Autodesk Inventor part; units mm, degrees
note: some values were not read from the file. Chosen so that the rebuilt part matches the saved one: direction of "Hole2".
(part 14 of 20)
  spline S82 degree 3 poles (-108.596575, -51.704661) (-108.591829, -51.705287) (-108.581504, -51.706647) (-108.566848, -51.71629) (-108.552275, -51.730819) (-108.537912, -51.751139) (-108.524031, -51.776791) (-108.505397, -51.819556) (-108.489595, -51.868576) (-108.475979, -51.923076) (-108.46262, -51.987447) (-108.449286, -52.075757) (-108.439921, -52.186978) (-108.436583, -52.301561) (-108.439921, -52.416145) (-108.449286, -52.527366) (-108.46262, -52.615676) (-108.475979, -52.680047) (-108.489595, -52.734547) (-108.505397, -52.783567) (-108.524031, -52.826332) (-108.537912, -52.851984) (-108.552275, -52.872304) (-108.566848, -52.886832) (-108.581504, -52.896476) (-108.591829, -52.897836) (-108.596575, -52.898461) knots 0 0 0 0 0.01106677 0.02407754 0.03992786 0.05913986 0.0819337 0.10802006 0.16805875 0.20201508 0.23929564 0.3216678 0.41056278 0.5 0.58943722 0.6783322 0.76070436 0.79798492 0.83194125 0.89197994 0.9180663 0.94086014 0.96007214 0.97592246 0.98893323 1 1 1 1
  spline S83 degree 3 poles (-108.596575, -52.898461) (-108.601237, -52.897852) (-108.611254, -52.896542) (-108.62517, -52.886862) (-108.638409, -52.872259) (-108.65094, -52.851903) (-108.662566, -52.826236) (-108.677691, -52.783344) (-108.689782, -52.734349) (-108.699832, -52.679969) (-108.709479, -52.61551) (-108.718735, -52.527157) (-108.725048, -52.416046) (-108.727236, -52.301561) (-108.725048, -52.187077) (-108.718735, -52.075966) (-108.709479, -51.987613) (-108.699832, -51.923154) (-108.689782, -51.868774) (-108.677691, -51.819779) (-108.662566, -51.776887) (-108.65094, -51.75122) (-108.638409, -51.730864) (-108.62517, -51.716261) (-108.611254, -51.706581) (-108.601237, -51.705271) (-108.596575, -51.704661) knots 0 0 0 0 0.01099744 0.02362844 0.03895388 0.0576141 0.07990846 0.10559498 0.1652091 0.19914929 0.2365432 0.31951534 0.40940333 0.5 0.59059667 0.68048466 0.7634568 0.80085071 0.8347909 0.89440502 0.92009154 0.9423859 0.96104612 0.97637156 0.98900256 1 1 1 1
  spline S84 degree 3 poles (-85.406507, -52.898461) (-85.411253, -52.897836) (-85.421579, -52.896476) (-85.436235, -52.886832) (-85.450807, -52.872304) (-85.46517, -52.851984) (-85.479051, -52.826332) (-85.497685, -52.783567) (-85.513487, -52.734547) (-85.527103, -52.680047) (-85.540462, -52.615676) (-85.553796, -52.527366) (-85.563161, -52.416145) (-85.566499, -52.301561) (-85.563161, -52.186978) (-85.553796, -52.075757) (-85.540462, -51.987447) (-85.527103, -51.923076) (-85.513487, -51.868576) (-85.497685, -51.819556) (-85.479051, -51.776791) (-85.46517, -51.751139) (-85.450807, -51.730819) (-85.436235, -51.71629) (-85.421579, -51.706647) (-85.411253, -51.705287) (-85.406507, -51.704661) knots 0 0 0 0 0.01106677 0.02407754 0.03992786 0.05913986 0.0819337 0.10802006 0.16805875 0.20201508 0.23929564 0.3216678 0.41056278 0.5 0.58943722 0.6783322 0.76070436 0.79798492 0.83194125 0.89197994 0.9180663 0.94086014 0.96007214 0.97592246 0.98893323 1 1 1 1
  spline S85 degree 3 poles (-85.406507, -51.704661) (-85.401845, -51.705271) (-85.391828, -51.706581) (-85.377912, -51.716261) (-85.364673, -51.730864) (-85.352142, -51.75122) (-85.340516, -51.776887) (-85.325391, -51.819779) (-85.3133, -51.868774) (-85.30325, -51.923154) (-85.293603, -51.987613) (-85.284347, -52.075966) (-85.278034, -52.187077) (-85.275846, -52.301561) (-85.278034, -52.416046) (-85.284347, -52.527157) (-85.293603, -52.61551) (-85.30325, -52.679969) (-85.3133, -52.734349) (-85.325391, -52.783344) (-85.340516, -52.826236) (-85.352142, -52.851903) (-85.364673, -52.872259) (-85.377912, -52.886862) (-85.391828, -52.896542) (-85.401845, -52.897852) (-85.406507, -52.898461) knots 0 0 0 0 0.01099744 0.02362844 0.03895388 0.0576141 0.07990846 0.10559498 0.1652091 0.19914929 0.2365432 0.31951534 0.40940333 0.5 0.59059667 0.68048466 0.7634568 0.80085071 0.8347909 0.89440502 0.92009154 0.9423859 0.96104612 0.97637156 0.98900256 1 1 1 1
  line L1833 (-101.214785, -54.709561) -> (-101.214785, -54.801561)
  line L1834 (-106.155772, -54.801561) -> (-106.155772, -54.201561)
  line L1835 (-101.214785, -54.801561) -> (-106.155772, -54.801561)
  line L1836 (-92.788297, -54.801561) -> (-92.788297, -54.709561)
  line L1837 (-87.84731, -54.801561) -> (-92.788297, -54.801561)
  line L1838 (-87.84731, -54.201561) -> (-87.84731, -54.801561)
  line L1839 (-101.001541, -54.201561) -> (-106.155772, -54.201561)
  line L1840 (-87.84731, -54.201561) -> (-93.001541, -54.201561)
  line L1841 (-85.051541, -54.801561) -> (-87.84731, -54.801561)
  line L1842 (-106.155772, -54.801561) -> (-108.951541, -54.801561)
  line L1843 (-93.001541, -49.801561) -> (-85.051541, -49.801561)
  line L1844 (-108.951541, -49.801561) -> (-101.001541, -49.801561)
  line L1845 (-108.951541, -54.801561) -> (-108.951541, -49.801561)
  line L1846 (-85.051541, -54.801561) -> (-85.051541, -49.801561)
  line L1847 (-92.788297, -54.801561) -> (-93.098156, -54.801561)
  line L1848 (-93.098156, -54.801561) -> (-93.098156, -54.709561)
  line L1849 (-93.098156, -54.801561) -> (-101.214785, -54.801561)
  line L1850 (-106.083905, -39.801561) -> (-100.326678, -39.801561)
  line L1851 (-93.676404, -39.801561) -> (-87.919177, -39.801561)
  line L1852 (-86.351309, -39.801561) -> (-85.788245, -39.801561)
  line L1853 (-108.214837, -39.801561) -> (-107.651773, -39.801561)
  line L1854 (-85.788245, -49.801561) -> (-85.788245, -39.801561)
  line L1855 (-108.214837, -39.801561) -> (-108.214837, -49.801561)
  spline S86 degree 3 poles (-105.769333, -47.200601) (-105.769074, -47.090365) (-105.765671, -46.866439) (-105.74757, -46.534003) (-105.717423, -46.260803) (-105.684088, -46.071483) (-105.649602, -45.979267) (-105.626193, -45.9168) (-105.576966, -45.914333) (-105.549364, -45.954376) (-105.514531, -46.034958) (-105.477403, -46.221178) (-105.445921, -46.494501) (-105.427985, -46.825972) (-105.423589, -47.159297) (-105.431148, -47.492218) (-105.451141, -47.826101) (-105.483037, -48.098141) (-105.518843, -48.287815) (-105.551255, -48.379074) (-105.575083, -48.444765) (-105.624435, -48.444965) (-105.650788, -48.40348) (-105.681562, -48.322842) (-105.718652, -48.137084) (-105.747883, -47.864653) (-105.76544, -47.532488) (-105.76959, -47.309883) (-105.769333, -47.200601) knots 0 0 0 0 0.06370705 0.12949472 0.19191208 0.22368799 0.2382902 0.25135028 0.25660425 0.26301775 0.27714857 0.30853838 0.37103998 0.43687849 0.50002298 0.56369496 0.62938323 0.69283553 0.72316052 0.73857311 0.75180992 0.75696152 0.7632602 0.77795176 0.80804313 0.87131401 0.93684349 1 1 1 1
  spline S87 degree 3 poles (-107.965507, -47.119008) (-107.964893, -46.896289) (-107.954528, -46.572436) (-107.954488, -46.176033) (-107.916737, -46.017933) (-107.925964, -45.924139) (-107.889328, -45.914097) (-107.8786, -45.994541) (-107.86006, -46.081863) (-107.845025, -46.30216) (-107.831555, -46.57198) (-107.82423, -46.905828) (-107.820159, -47.352241) (-107.835826, -47.785121) (-107.839355, -48.182231) (-107.879062, -48.341118) (-107.869754, -48.435677) (-107.907095, -48.446175) (-107.915715, -48.363737) (-107.933723, -48.276705) (-107.945951, -48.0556) (-107.962013, -47.678267) (-107.966123, -47.341986) (-107.965507, -47.119008) knots 0 0 0 0 0.13139199 0.19506211 0.22486648 0.236537 0.23877104 0.24363774 0.27264718 0.30298792 0.36807806 0.43503205 0.49911295 0.63103815 0.69471519 0.72474683 0.73665002 0.73889428 0.74387281 0.77307947 0.80345172 0.86845517 1 1 1 1
  spline S88 degree 3 poles (-88.577615, -47.119008) (-88.57729, -47.008677) (-88.574234, -46.78406) (-88.552396, -46.455188) (-88.522944, -46.174531) (-88.475521, -46.007946) (-88.439428, -45.916086) (-88.390424, -45.914818) (-88.347089, -45.976964) (-88.316595, -46.08799) (-88.279777, -46.300167) (-88.252588, -46.57628) (-88.236182, -46.907606) (-88.231986, -47.240889) (-88.239004, -47.574267) (-88.258558, -47.903462) (-88.289101, -48.183006) (-88.332842, -48.350609) (-88.365074, -48.442504) (-88.414556, -48.446229) (-88.458229, -48.380683) (-88.485965, -48.271583) (-88.527334, -48.059183) (-88.5545, -47.78425) (-88.573579, -47.45108) (-88.577937, -47.228226) (-88.577615, -47.119008) knots 0 0 0 0 0.06377364 0.12947571 0.19191728 0.22251596 0.23572674 0.24098241 0.24712107 0.27642984 0.3084167 0.37100213 0.43691035 0.50001881 0.5637377 0.62924964 0.69193924 0.72212339 0.73538665 0.74053978 0.7469427 0.77702751 0.80721947 0.87118814 0.93686953 1 1 1 1
  line L1856 (-87.919177, -39.801561) -> (-86.351309, -39.801561)
  line L1857 (-107.651773, -39.801561) -> (-106.083905, -39.801561)
  spline S89 degree 3 poles (-86.180316, -47.200601) (-86.179625, -46.976697) (-86.177708, -46.642662) (-86.153357, -46.263675) (-86.144704, -46.070685) (-86.121116, -45.985378) (-86.127644, -45.919582) (-86.090265, -45.91624) (-86.086845, -45.961563) (-86.067375, -46.033845) (-86.058579, -46.22558) (-86.044067, -46.494224) (-86.038541, -46.826549) (-86.036712, -47.27203) (-86.040139, -47.717725) (-86.061167, -48.094625) (-86.068571, -48.289359) (-86.090145, -48.371714) (-86.082612, -48.443355) (-86.120246, -48.442499) (-86.123349, -48.396914) (-86.142857, -48.32401) (-86.154386, -48.133195) (-86.177012, -47.757195) (-86.181004, -47.423111) (-86.180316, -47.200601) knots 0 0 0 0 0.13209168 0.19547472 0.22735918 0.24158397 0.25296859 0.25518606 0.26025608 0.27356013 0.30485536 0.36824052 0.43535326 0.4998067 0.63172546 0.69607433 0.72644443 0.74148548 0.75299654 0.75519516 0.76033444 0.77439415 0.80449955 0.86873005 1 1 1 1
  line L1858 (-93.001541, -42.271561) -> (-95.001541, -34.951561)
  line L1859 (-99.001541, -34.951561) -> (-101.001541, -42.271561)
  line L1860 (-93.001541, -53.693561) -> (-93.001541, -42.271561)
  line L1861 (-101.001541, -53.693561) -> (-101.001541, -42.271561)
  line L1862 (-95.001541, -34.951561) -> (-99.001541, -34.951561)
  line L1863 (-93.001541, -53.693561) -> (-93.001541, -54.709561)
  line L1864 (-101.001541, -53.693561) -> (-101.001541, -54.709561)
  line L1865 (-93.001541, -54.709561) -> (-101.001541, -54.709561)
  line L1866 (-105.126509, -54.709561) -> (-105.301369, -54.709561)
  line L1867 (-105.126509, -54.201561) -> (-105.126509, -54.709561)
  line L1868 (-101.424102, -54.709561) -> (-105.126509, -54.709561)
  line L1869 (-101.424102, -54.709561) -> (-101.001541, -54.709561)
  line L1870 (-93.001541, -54.709561) -> (-92.57898, -54.709561)
  line L1871 (-88.876573, -54.709561) -> (-92.57898, -54.709561)
  line L1872 (-88.876573, -54.201561) -> (-88.876573, -54.709561)
  line L1873 (-88.701713, -54.709561) -> (-88.876573, -54.709561)
  line L1874 (-105.301369, -54.201561) -> (-105.301369, -54.709561)
  line L1875 (-88.701713, -54.201561) -> (-88.701713, -54.709561)
  line L1876 (-108.001541, -57.801561) -> (-86.001541, -57.801561)
  line L1877 (-108.001541, -90.801561) -> (-86.001541, -90.801561)
  line L1878 (-108.001541, -90.801561) -> (-108.001541, -57.801561)
  line L1879 (-86.001541, -90.801561) -> (-86.001541, -57.801561)
  line L1880 (-106.400026, -57.801561) -> (-106.400026, -54.801561)
  line L1881 (-104.300026, -57.801561) -> (-104.300026, -54.801561)
  line L1882 (-98.051541, -57.801561) -> (-98.051541, -54.801561)
  line L1883 (-95.951541, -57.801561) -> (-95.951541, -54.801561)
  line L1884 (-89.703056, -57.801561) -> (-89.703056, -54.801561)
  line L1885 (-87.603056, -57.801561) -> (-87.603056, -54.801561)
  point P0 (0, 0)
sketch "Sketch13" plane through (0, 0, 0) normal (1, 0, 0) x (0, 1, 0)
  line L0 (0, -156.78708) -> (0, 91.844197)
  line L1 (0, 25) -> (0, -118.976908)
  line L2 (13.762, 0) -> (-13.762, 0)
  line L3 (-13.762, -15) -> (-13.762, 0)
  line L4 (-0.000559, -82.705424) -> (-0.000559, -41.705424)
  line L5 (6.538534, -24.585438) -> (6.563068, -24.580402)
  ellipse E0 centre (6.661555, -24.562642) end of major axis (7.445275, -24.402071) minor radius 0.002388 (6.818055, -24.52819) -> (6.563068, -24.580402) ccw
  ellipse E1 centre (6.661555, -24.562642) end of major axis (7.445275, -24.402071) minor radius 0.002388 (7.445275, -24.402071) -> (6.993202, -24.492485) ccw
  line L6 (7.445414, -24.402746) -> (7.445275, -24.402071)
  ellipse E2 centre (-6.654323, -24.56163) end of major axis (-7.438018, -24.400939) minor radius 0.002388 (-6.987316, -24.491146) -> (-7.438018, -24.400939) ccw
  line L7 (-5.641341, -24.766384) -> (-5.408876, -24.813938)
  line L8 (-7.438157, -24.401614) -> (-7.438018, -24.400939)
  ellipse E3 centre (6.129182, -24.706286) end of major axis (6.887302, -24.450836) minor radius 0.00228 (6.197609, -24.680834) -> (6.046176, -24.731863) ccw
  ellipse E4 centre (6.129182, -24.706286) end of major axis (6.887302, -24.450836) minor radius 0.00228 (6.315844, -24.641059) -> (6.203449, -24.678867) ccw
  ellipse E5 centre (6.129182, -24.706286) end of major axis (6.887302, -24.450836) minor radius 0.00228 (6.887302, -24.450836) -> (6.7158, -24.507102) ccw
  line L9 (6.890035, -24.458948) -> (6.887302, -24.450836)
  line L10 (4.330668, -24.56025) -> (2.677597, -19.654302)
  ellipse E6 centre (8.77147, -25.619916) end of major axis (7.994045, -25.808624) minor radius 0.136933 (8.476682, -25.558962) -> (8.459659, -25.56427) ccw
  line L11 (8.188929, -25.631093) -> (8.37952, -25.5808)
  ellipse E7 centre (9.003874, -26.577355) end of major axis (8.517983, -26.695298) minor radius 0.085583 (8.8835, -26.520415) -> (8.736952, -26.713693) ccw
  ellipse E8 centre (-9.68688, -24.534712) end of major axis (-10.486627, -24.554802) minor radius 0.133925 (-10.038142, -24.422936) -> (-10.486627, -24.554802) ccw
  line L12 (-9.713956, -24.401484) -> (-8.140476, -24.354137)
  line L13 (-8.140476, -24.354137) -> (-8.135518, -24.551512)
  ellipse E9 centre (-9.637363, -26.505866) end of major axis (-10.43711, -26.525957) minor radius 0.133925 (-9.365334, -26.373246) -> (-9.664439, -26.372638) ccw
  line L14 (-8.140476, -24.354137) -> (-8.15036, -23.96069)
  line L15 (-8.167314, -23.285776) -> (-8.191572, -22.320133)
  ellipse E10 centre (-10.031023, -10.83519) end of major axis (-12.120364, -10.887676) minor radius 0.349879 (-10.885047, -10.536629) -> (-11.139823, -10.565627) ccw
  ellipse E11 centre (-10.00874, -11.72221) end of major axis (-12.098081, -11.774696) minor radius 0.349879 (-10.871432, -11.424514) -> (-11.106976, -11.451287) ccw
  ellipse E12 centre (-10.00874, -11.72221) end of major axis (-11.508267, -11.759879) minor radius 0.251109 (-9.215053, -11.489714) -> (-11.464502, -11.818006) ccw
  ellipse E13 centre (-9.637363, -26.505866) end of major axis (-10.137205, -26.518423) minor radius 0.083703 (-9.71107, -26.424853) -> (-9.885839, -26.584584) ccw
  ellipse E14 centre (-7.235042, -24.481629) end of major axis (-8.032995, -24.424433) minor radius 0.002347 (-7.349169, -24.47112) -> (-8.032995, -24.424433) ccw
  line L16 (-7.349169, -24.47112) -> (-7.290502, -24.4753)
  line L17 (-7.053927, -24.492157) -> (-5.794483, -24.581895)
  line L18 (-5.794483, -24.581895) -> (-5.809794, -24.7955)
  line L19 (-8.03394, -24.43762) -> (-8.032995, -24.424433)
  line L20 (-5.794483, -24.581895) -> (-5.675138, -22.916899)
  line L21 (6.124958, -24.147667) -> (6.192678, -24.489837)
  line L22 (5.156701, -24.971123) -> (6.630008, -24.699822)
  ellipse E15 centre (6.697382, -24.588787) end of major axis (7.48216, -24.433469) minor radius 0.096422 (6.630008, -24.699822) -> (7.339309, -24.407098) ccw
  line L23 (7.339309, -24.407098) -> (6.817508, -24.416015)
  line L24 (7.483693, -24.441211) -> (7.48216, -24.433469)
  line L25 (8.639126, -24.265814) -> (8.649991, -24.369649)
  line L26 (8.133427, -24.573507) -> (9.009078, -24.476939)
  ellipse E16 centre (9.115563, -24.49988) end of major axis (9.911219, -24.416622) minor radius 0.034185 (9.875937, -24.410338) -> (9.009078, -24.476939) ccw
  ellipse E17 centre (7.670285, -10.687987) end of major axis (9.748936, -10.470477) minor radius 0.089309 (9.606621, -10.453086) -> (9.105415, -10.473132) ccw
  ellipse E18 centre (7.763864, -11.582283) end of major axis (9.842515, -11.364772) minor radius 0.089309 (9.697526, -11.347367) -> (9.630114, -11.347814) ccw
  ellipse E19 centre (9.323517, -26.487202) end of major axis (8.826232, -26.539238) minor radius 0.021366 (8.947051, -26.512487) -> (8.849644, -26.530183) ccw
  ellipse E20 centre (9.323517, -26.487202) end of major axis (9.820802, -26.435166) minor radius 0.021366 (9.780884, -26.430998) -> (9.511362, -26.447692) ccw
  ellipse E21 centre (-3.296494, -25.822087) end of major axis (-2.590337, -25.968059) minor radius 0.431228 (-4.004737, -25.771436) -> (-3.988038, -25.8345) ccw
  line L27 (-7.692462, -23.876411) -> (-7.75112, -24.436159)
  ellipse E22 centre (-9.108321, -24.498494) end of major axis (-8.312678, -24.581872) minor radius 0.034185 (-9.138885, -24.46095) -> (-9.8417, -24.408452) ccw
  line L28 (-9.138885, -24.46095) -> (-8.125826, -24.565234)
  line L29 (-7.555939, -24.452228) -> (-7.496702, -23.886955)
  ellipse E23 centre (-7.660942, -10.686822) end of major axis (-9.73956, -10.468995) minor radius 0.089309 (-9.096039, -10.471748) -> (-9.597242, -10.451626) ccw
  ellipse E24 centre (-7.754657, -11.581103) end of major axis (-9.833275, -11.363276) minor radius 0.089309 (-9.620871, -11.34635) -> (-9.688283, -11.345892) ccw
  ellipse E25 centre (-7.754657, -11.581103) end of major axis (-9.246488, -11.424768) minor radius 0.064098 (-9.206248, -11.414395) -> (-9.20961, -11.443158) ccw
  ellipse E26 centre (-9.316577, -26.485785) end of major axis (-8.8193, -26.537896) minor radius 0.021366 (-8.850179, -26.542023) -> (-8.940115, -26.511127) ccw
  ellipse E27 centre (-9.316577, -26.485785) end of major axis (-9.813854, -26.433673) minor radius 0.021366 (-9.504416, -26.446246) -> (-9.782585, -26.444538) ccw
  line L30 (-4.820661, -21.84423) -> (-5.420588, -24.873067)
  line L31 (-7.12486, -24.420134) -> (-7.202788, -24.413344)
  ellipse E28 centre (-6.690154, -24.587769) end of major axis (-7.474908, -24.432331) minor radius 0.096422 (-7.202788, -24.413344) -> (-6.815159, -24.660395) ccw
  line L32 (-6.815159, -24.660395) -> (-5.289587, -24.988815)
  line L33 (-5.289587, -24.988815) -> (-5.298773, -25.035191)
  line L34 (-7.476442, -24.440074) -> (-7.474908, -24.432331)
  line L35 (-5.344977, -24.953512) -> (-5.289587, -24.988815)
  line L36 (-5.289587, -24.988815) -> (-4.670217, -21.861819)
  line L37 (6.992718, -24.498291) -> (7.160798, -24.486218)
  ellipse E29 centre (7.242286, -24.48273) end of major axis (8.040248, -24.425656) minor radius 0.002347 (8.040248, -24.425656) -> (7.160798, -24.486218) ccw
  line L38 (8.041191, -24.438842) -> (8.040248, -24.425656)
  line L39 (5.397246, -21.789513) -> (5.396468, -21.778626)
  line L40 (9.270678, -24.196238) -> (9.265813, -24.388739)
  line L41 (8.05276, -24.399003) -> (9.583486, -24.40079)
  ellipse E30 centre (9.694116, -24.536186) end of major axis (10.493861, -24.556398) minor radius 0.133925 (10.493861, -24.556398) -> (9.583486, -24.40079) ccw
  ellipse E31 centre (10.040343, -10.836717) end of major axis (7.95101, -10.783913) minor radius 0.349879 (11.149184, -10.567322) -> (10.894413, -10.538285) ccw
  ellipse E32 centre (10.017925, -11.723733) end of major axis (7.928593, -11.670929) minor radius 0.349879 (11.116202, -11.452978) -> (10.880662, -11.426168) ccw
  ellipse E33 centre (10.017925, -11.723733) end of major axis (11.517447, -11.76163) minor radius 0.251109 (11.453613, -11.831515) -> (9.224274, -11.491116) ccw
  ellipse E34 centre (9.669208, -25.521759) end of major axis (8.869463, -25.501547) minor radius 0.133925 (9.558577, -25.386363) -> (9.538557, -25.386383) ccw
  ellipse E35 centre (9.644299, -26.507333) end of major axis (9.144459, -26.4947) minor radius 0.083703 (9.892763, -26.586088) -> (9.915942, -26.584291) ccw
  ellipse E36 centre (9.644299, -26.507333) end of major axis (10.14414, -26.519965) minor radius 0.083703 (9.969198, -26.451685) -> (9.718019, -26.42633) ccw
  line L42 (-8.295321, -25.586863) -> (-8.180997, -25.613451)
  ellipse E37 centre (-8.764398, -25.618582) end of major axis (-9.541794, -25.429755) minor radius 0.136933 (-8.452579, -25.562984) -> (-8.471155, -25.557192) ccw
  ellipse E38 centre (-8.996948, -26.575986) end of major axis (-8.511075, -26.694003) minor radius 0.085583 (-8.730047, -26.712365) -> (-8.876566, -26.519064) ccw
  ellipse E39 centre (-6.121972, -24.705355) end of major axis (-6.880052, -24.449789) minor radius 0.00228 (-6.709864, -24.505646) -> (-6.880052, -24.449789) ccw
  line L43 (-4.902478, -25.65651) -> (-5.057548, -26.116494)
  line L44 (-6.882787, -24.4579) -> (-6.880052, -24.449789)
  line L45 (-3.997314, -22.971536) -> (-2.763273, -19.311016)
  line L46 (-4.81826, -25.990761) -> (-5.057548, -26.116494)
  line L47 (-5.057548, -26.116494) -> (-5.080907, -26.108852)
  line L48 (-5.380616, -26.007714) -> (-5.057548, -26.116494)
  line L49 (6.357957, -24.626653) -> (6.513804, -24.592143)
  ellipse E40 centre (6.593486, -24.577142) end of major axis (7.374623, -24.40444) minor radius 0.002568 (6.642154, -24.563757) -> (6.513804, -24.592143) ccw
  ellipse E41 centre (6.593486, -24.577142) end of major axis (7.374623, -24.40444) minor radius 0.002568 (6.758444, -24.538101) -> (6.645183, -24.563088) ccw
  ellipse E42 centre (6.593486, -24.577142) end of major axis (7.374623, -24.40444) minor radius 0.002568 (7.374623, -24.40444) -> (6.957315, -24.494376) ccw
  line L50 (7.375071, -24.406468) -> (7.374623, -24.40444)
  ellipse E43 centre (9.322809, -26.624245) end of major axis (10.117918, -26.535923) minor radius 0.263102 (8.636355, -26.825912) -> (8.782558, -26.871903) ccw
  ellipse E44 centre (9.322809, -26.624245) end of major axis (10.117918, -26.535923) minor radius 0.263102 (9.884151, -26.756187) -> (10.048681, -26.66076) ccw
  ellipse E45 centre (-9.31589, -26.622828) end of major axis (-10.110986, -26.534385) minor radius 0.263102 (-9.845155, -26.372868) -> (-9.996156, -26.418233) ccw
  ellipse E46 centre (-9.31589, -26.622828) end of major axis (-10.110986, -26.534385) minor radius 0.263102 (-10.02645, -26.433412) -> (-10.035402, -26.438628) ccw
  ellipse E47 centre (-9.31589, -26.622828) end of major axis (-10.110986, -26.534385) minor radius 0.263102 (-10.102006, -26.585729) -> (-9.877252, -26.754684) ccw
  ellipse E48 centre (-9.31589, -26.622828) end of major axis (-8.520794, -26.711271) minor radius 0.263102 (-8.775677, -26.870568) -> (-8.629467, -26.824599) ccw
  line L51 (4.409189, -25.366587) -> (4.528129, -25.320401)
  ellipse E49 centre (5.938789, -24.775263) end of major axis (6.684616, -24.485881) minor radius 0.002457 (6.060507, -24.725437) -> (6.044004, -24.731831) ccw
  ellipse E50 centre (5.938789, -24.775263) end of major axis (6.684616, -24.485881) minor radius 0.002457 (6.154843, -24.688912) -> (6.106425, -24.707653) ccw
  ellipse E51 centre (5.938789, -24.775263) end of major axis (6.684616, -24.485881) minor radius 0.002457 (6.684616, -24.485881) -> (6.613079, -24.512514) ccw
  line L52 (4.770915, -26.298867) -> (4.409189, -25.366587)
  ellipse E52 centre (6.66224, -26.639822) end of major axis (5.916413, -26.929204) minor radius 0.002457 (6.36138, -26.754143) -> (6.371729, -26.754967) ccw
  line L53 (5.916413, -26.929204) -> (5.554687, -25.996924)
  line L54 (6.690509, -24.501071) -> (6.684616, -24.485881)
  line L55 (4.409189, -25.366587) -> (2.477246, -20.38737)
  line L56 (5.555569, -25.999197) -> (4.770915, -26.298867)
  line L57 (4.770915, -26.298867) -> (4.420552, -26.113515)
  ellipse E53 centre (4.748342, -25.988327) end of major axis (3.873588, -25.603559) minor radius 0.25544 (3.876642, -25.676845) -> (4.420552, -26.113515) ccw
  line L58 (3.876642, -25.676845) -> (2.376118, -21.809529)
  ellipse E54 centre (6.300514, -25.707543) end of major axis (5.554687, -25.996924) minor radius 0.002457 (5.701086, -25.938551) -> (5.554687, -25.996924) ccw
  line L59 (4.770915, -26.298867) -> (5.69639, -25.939489)
  ellipse E55 centre (6.66224, -26.639822) end of major axis (6.196098, -26.820686) minor radius 0.001536 (6.363795, -26.754353) -> (6.369241, -26.754786) ccw
  ellipse E56 centre (8.632199, -25.664331) end of major axis (7.863499, -25.885917) minor radius 0.14613 (8.422512, -25.576471) -> (8.190586, -25.662652) ccw
  line L60 (8.189685, -25.645493) -> (8.414784, -25.577173)
  ellipse E57 centre (8.904521, -26.60904) end of major axis (8.424084, -26.747532) minor radius 0.091331 (8.881254, -26.520698) -> (8.745355, -26.742842) ccw
  ellipse E58 centre (8.904521, -26.60904) end of major axis (8.135821, -26.830626) minor radius 0.14613 (8.577328, -26.562491) -> (8.636355, -26.825912) ccw
  line L61 (8.135821, -26.830626) -> (8.024756, -26.445332)
  line L62 (0.609327, -23.619508) -> (0.581005, -23.162788)
  line L63 (-4.476077, -26.044132) -> (-4.398814, -26.180209)
  line L64 (-4.398814, -26.180209) -> (-3.921996, -26.073355)
  ellipse E59 centre (-2.644242, -26.591909) end of major axis (-3.417521, -26.796945) minor radius 0.142054 (-3.417521, -26.796945) -> (-2.999871, -26.813423) ccw
  line L65 (-3.417521, -26.796945) -> (-3.592587, -26.1367)
  line L66 (-9.196668, -24.374978) -> (-9.205417, -24.201661)
  line L67 (-8.449337, -24.27744) -> (-8.446285, -24.337908)
  ellipse E60 centre (-9.798412, -24.547864) end of major axis (-10.597394, -24.588197) minor radius 0.142983 (-10.081083, -24.427776) -> (-10.597394, -24.588197) ccw
  line L68 (-9.800805, -24.404823) -> (-8.227885, -24.327119)
  line L69 (-8.227885, -24.327119) -> (-8.226391, -24.356722)
  ellipse E61 centre (-9.699202, -26.513159) end of major axis (-10.498185, -26.553492) minor radius 0.142983 (-10.018984, -26.397591) -> (-10.041768, -26.659232) ccw
  ellipse E62 centre (-9.699202, -26.513159) end of major axis (-10.498185, -26.553492) minor radius 0.142983 (-9.428407, -26.36524) -> (-9.701595, -26.370117) ccw
  line L70 (-10.498185, -26.553492) -> (-10.597394, -24.588197)
  line L71 (-8.227885, -24.327119) -> (-8.229655, -24.292058)
  line L72 (-8.281282, -23.26936) -> (-8.322726, -22.448358)
  line L73 (-9.415067, -24.385767) -> (-9.425698, -24.17518)
  ellipse E63 centre (-10.487916, -10.889069) end of major axis (-12.575258, -10.994439) minor radius 0.373543 (-11.139823, -10.565627) -> (-12.575258, -10.994439) ccw
  ellipse E64 centre (-10.443272, -11.773451) end of major axis (-12.530614, -11.878821) minor radius 0.373543 (-11.106976, -11.451287) -> (-12.077988, -12.085909) ccw
  line L74 (-12.575258, -10.994439) -> (-12.530614, -11.878821)
  ellipse E65 centre (-10.443272, -11.773451) end of major axis (-11.941364, -11.849076) minor radius 0.268093 (-9.223048, -11.558091) -> (-11.785623, -11.958236) ccw
  ellipse E66 centre (-9.699202, -26.513159) end of major axis (-10.198566, -26.538367) minor radius 0.089364 (-9.714744, -26.424487) -> (-9.884793, -26.605293) ccw
  line L75 (-6.561399, -24.456113) -> (-6.538759, -24.025962)
  line L76 (-5.922911, -22.889104) -> (-5.933137, -23.083406)
  line L77 (-5.986476, -24.096822) -> (-6.009919, -24.542227)
  ellipse E67 centre (-7.320041, -24.476351) end of major axis (-8.118935, -24.434303) minor radius 0.002573 (-7.410997, -24.469003) -> (-8.118935, -24.434303) ccw
  line L78 (-7.410997, -24.469003) -> (-5.848535, -24.550661)
  line L79 (-5.848535, -24.550661) -> (-5.849971, -24.577941)
  ellipse E68 centre (-7.42516, -26.473576) end of major axis (-8.224054, -26.431528) minor radius 0.002573 (-7.762294, -26.453495) -> (-7.752898, -26.458677) ccw
  line L80 (-8.224054, -26.431528) -> (-8.118935, -24.434303)
  line L81 (-5.848535, -24.550661) -> (-5.762145, -22.909285)
  line L82 (-6.722685, -24.445814) -> (-6.710298, -24.210463)
  ellipse E69 centre (-7.42516, -26.473576) end of major axis (-7.924469, -26.447296) minor radius 0.001608 (-7.760051, -26.454755) -> (-7.755232, -26.457412) ccw
  line L83 (5.199521, -24.469687) -> (4.647875, -21.866031)
  ellipse E70 centre (6.642771, -24.619059) end of major axis (8.012367, -24.328877) minor radius 0.211294 (6.095158, -24.534439) -> (6.071274, -24.541062) ccw
  line L84 (6.018037, -24.170443) -> (6.095158, -24.534439)
  line L85 (5.067297, -25.057107) -> (5.163856, -25.008007)
  line L86 (6.095158, -24.534439) -> (6.171698, -24.495518)
  line L87 (5.067297, -25.057107) -> (6.607154, -24.749655)
  ellipse E71 centre (6.642771, -24.619059) end of major axis (7.425397, -24.453241) minor radius 0.120739 (6.607154, -24.749655) -> (7.264342, -24.415474) ccw
  line L88 (7.264342, -24.415474) -> (6.348163, -24.416584)
  line L89 (5.272196, -26.024184) -> (5.067297, -25.057107)
  ellipse E72 centre (7.052568, -26.553214) end of major axis (6.269941, -26.719032) minor radius 0.120739 (6.36138, -26.754143) -> (7.769239, -26.454677) ccw
  line L90 (7.427064, -24.461109) -> (7.425397, -24.453241)
  line L91 (5.067297, -25.057107) -> (4.396393, -21.890579)
  line L92 (5.272196, -26.024184) -> (4.950446, -25.766483)
  ellipse E73 centre (5.267606, -25.605207) end of major axis (4.474045, -25.039824) minor radius 0.319988 (4.457859, -25.160563) -> (4.950446, -25.766483) ccw
  line L93 (4.457859, -25.160563) -> (3.131339, -18.899671)
  line L94 (5.272196, -26.024184) -> (6.812052, -25.716732)
  line L95 (7.680029, -24.443744) -> (7.616727, -23.882065)
  line L96 (8.553941, -24.27428) -> (8.56439, -24.366996)
  line L97 (8.134393, -24.591902) -> (9.003472, -24.492195)
  ellipse E74 centre (9.079697, -24.500677) end of major axis (9.874664, -24.411084) minor radius 0.01704 (9.861978, -24.409502) -> (9.003472, -24.492195) ccw
  ellipse E75 centre (9.303631, -26.487645) end of major axis (8.508663, -26.577239) minor radius 0.01704 (10.025937, -26.399115) -> (8.577328, -26.562491) ccw
  line L98 (7.415525, -24.402989) -> (7.358366, -23.895815)
  ellipse E76 centre (7.523357, -10.691255) end of major axis (9.600209, -10.457191) minor radius 0.044517 (9.531981, -10.453596) -> (9.106672, -10.483904) ccw
  ellipse E77 centre (7.624127, -11.58539) end of major axis (9.700979, -11.351326) minor radius 0.044517 (9.630114, -11.347814) -> (9.211035, -11.377726) ccw
  ellipse E78 centre (9.191664, -25.494161) end of major axis (8.396696, -25.583755) minor radius 0.01704 (9.115439, -25.485679) -> (8.422512, -25.576471) ccw
  line L99 (8.186889, -25.592209) -> (9.115439, -25.485679)
  ellipse E79 centre (9.303631, -26.487645) end of major axis (8.806776, -26.543641) minor radius 0.01065 (9.778165, -26.431012) -> (8.81437, -26.540893) ccw
  line L100 (1.583112, -23.619582) -> (1.632842, -23.162868)
  line L101 (3.67046, -25.515464) -> (2.519787, -25.509102)
  line L102 (2.678293, -26.089407) -> (3.990346, -26.096661)
  line L103 (3.990346, -26.096661) -> (4.096475, -25.923419)
  ellipse E80 centre (3.422826, -25.919695) end of major axis (4.134478, -25.73546) minor radius 0.371687 (3.81855, -25.527124) -> (3.67046, -25.515464) ccw
  ellipse E81 centre (3.422826, -25.919695) end of major axis (4.134478, -25.73546) minor radius 0.371687 (4.096475, -25.923419) -> (4.101148, -25.915584) ccw
  ellipse E82 centre (2.276225, -26.634633) end of major axis (3.071524, -26.721231) minor radius 0.273562 (2.891037, -26.868283) -> (3.006761, -26.81388) ccw
  line L104 (-1.41197, -23.619354) -> (-1.461632, -23.162633)
  ellipse E83 centre (-3.272029, -25.943789) end of major axis (-2.564265, -26.037032) minor radius 0.400382 (-3.439222, -25.537366) -> (-3.961747, -25.976725) ccw
  line L105 (-3.980348, -25.905222) -> (-3.995625, -25.764726)
  line L106 (-2.508379, -25.492916) -> (-3.439222, -25.537366)
  line L107 (-3.961747, -25.976725) -> (-3.890093, -26.150907)
  line L108 (-3.890093, -26.150907) -> (-2.672319, -26.092755)
  ellipse E84 centre (-2.269308, -26.634287) end of major axis (-3.06462, -26.720765) minor radius 0.273562 (-2.999871, -26.813423) -> (-2.884155, -26.867844) ccw
  ellipse E85 centre (-9.072455, -24.499297) end of major axis (-9.867409, -24.409582) minor radius 0.01704 (-9.078165, -24.481505) -> (-9.854723, -24.408003) ccw
  line L109 (-9.078165, -24.481505) -> (-8.127058, -24.588646)
  ellipse E86 centre (-9.296691, -26.48623) end of major axis (-10.091645, -26.396515) minor radius 0.01704 (-8.5704, -26.561187) -> (-10.018984, -26.397591) ccw
  line L110 (-7.48462, -24.403923) -> (-7.426698, -23.890685)
  ellipse E87 centre (-7.514015, -10.690111) end of major axis (-9.590831, -10.455732) minor radius 0.044517 (-9.097299, -10.482519) -> (-9.590831, -10.455732) ccw
  ellipse E88 centre (-7.614921, -11.584231) end of major axis (-9.691737, -11.349851) minor radius 0.044517 (-9.201797, -11.376326) -> (-9.620871, -11.34635) ccw
  line L111 (-9.190283, -25.474972) -> (-8.1797, -25.588813)
  ellipse E89 centre (-9.184573, -25.492764) end of major axis (-8.389619, -25.582478) minor radius 0.01704 (-8.415434, -25.57519) -> (-9.190283, -25.474972) ccw
  ellipse E90 centre (-9.296691, -26.48623) end of major axis (-9.793537, -26.430158) minor radius 0.01065 (-8.853118, -26.541095) -> (-9.745466, -26.440206) ccw
  line L112 (-6.177395, -24.480632) -> (-7.162076, -24.417758)
  ellipse E91 centre (-6.635547, -24.618049) end of major axis (-7.418148, -24.452112) minor radius 0.120739 (-7.162076, -24.417758) -> (-6.740176, -24.718646) ccw
  line L113 (-6.740176, -24.718646) -> (-5.212596, -25.067292)
  line L114 (-5.212596, -25.067292) -> (-5.417642, -26.034338)
  ellipse E92 centre (-7.045638, -26.552142) end of major axis (-7.828239, -26.386204) minor radius 0.120739 (-7.762294, -26.453495) -> (-6.354481, -26.753176) ccw
  line L115 (-7.419817, -24.45998) -> (-7.418148, -24.452112)
  line L116 (-5.245364, -25.043922) -> (-5.212596, -25.067292)
  line L117 (-5.212596, -25.067292) -> (-4.536252, -21.877481)
  ellipse E93 centre (-5.279378, -25.643299) end of major axis (-4.46703, -25.084437) minor radius 0.235923 (-5.075768, -25.788508) -> (-4.467316, -25.176997) ccw
  line L118 (-4.399469, -24.868199) -> (-3.14654, -18.959069)
  line L119 (-5.075768, -25.788508) -> (-5.417642, -26.034338)
  line L120 (-6.945221, -25.685692) -> (-5.417642, -26.034338)
  line L121 (5.951048, -24.547397) -> (5.928252, -24.113016)
  line L122 (6.774387, -24.133897) -> (6.789194, -24.41605)
  line L123 (5.705778, -24.56032) -> (7.275122, -24.477631)
  ellipse E94 centre (7.327286, -24.477465) end of major axis (8.126187, -24.435538) minor radius 0.002573 (8.126187, -24.435538) -> (7.275122, -24.477631) ccw
  line L124 (5.708365, -24.609626) -> (5.705778, -24.56032)
  ellipse E95 centre (7.432101, -26.474706) end of major axis (8.231002, -26.432779) minor radius 0.002573 (7.759841, -26.459856) -> (7.769239, -26.454677) ccw
  line L125 (8.231002, -26.432779) -> (8.126187, -24.435538)
  line L126 (7.034946, -24.4123) -> (7.019422, -24.116489)
  line L127 (5.705778, -24.56032) -> (5.619759, -22.92126)
  ellipse E96 centre (7.432101, -26.474706) end of major axis (7.931414, -26.448502) minor radius 0.001608 (7.762176, -26.458592) -> (7.766995, -26.455936) ccw
  line L128 (8.425757, -24.362698) -> (8.4297, -24.284823)
  line L129 (9.346779, -24.187138) -> (9.33646, -24.390929)
  line L130 (8.160696, -24.354482) -> (9.725722, -24.402996)
  ellipse E97 centre (9.805646, -24.549355) end of major axis (10.604622, -24.58981) minor radius 0.142983 (10.604622, -24.58981) -> (10.088335, -24.429309) ccw
  line L131 (8.158436, -24.399126) -> (8.160696, -24.354482)
  ellipse E98 centre (9.706138, -26.514634) end of major axis (10.505114, -26.555089) minor radius 0.142983 (10.366012, -26.627699) -> (10.025937, -26.399115) ccw
  line L132 (10.505114, -26.555089) -> (10.604622, -24.58981)
  line L133 (9.601521, -24.399146) -> (9.613954, -24.153592)
  line L134 (8.160696, -24.354482) -> (8.170631, -24.15827)
  line L135 (8.250637, -22.578158) -> (8.263336, -22.327348)
  ellipse E99 centre (10.497228, -10.890665) end of major axis (12.584554, -10.996352) minor radius 0.373543 (12.584554, -10.996352) -> (11.149184, -10.567322) ccw
  ellipse E100 centre (10.452449, -11.77504) end of major axis (12.539775, -11.880728) minor radius 0.373543 (12.150312, -12.075826) -> (11.116202, -11.452978) ccw
  line L136 (12.584554, -10.996352) -> (12.539775, -11.880728)
  ellipse E101 centre (10.452449, -11.77504) end of major axis (11.95053, -11.850893) minor radius 0.268093 (11.807976, -11.955779) -> (9.232258, -11.559495) ccw
  ellipse E102 centre (9.706138, -26.514634) end of major axis (10.205498, -26.539919) minor radius 0.089364 (9.891715, -26.606797) -> (9.721693, -26.425965) ccw
  line L137 (4.006136, -26.070886) -> (4.491136, -26.168235)
  line L138 (4.491136, -26.168235) -> (4.500417, -26.155765)
  ellipse E103 centre (2.651166, -26.592311) end of major axis (3.424413, -26.797466) minor radius 0.142054 (3.006761, -26.81388) -> (3.424413, -26.797466) ccw
  line L139 (3.424413, -26.797466) -> (3.610904, -26.094563)
  line L140 (-0.444929, -23.619428) -> (-0.416537, -23.162712)
  line L141 (-8.390893, -25.577423) -> (-8.182211, -25.636517)
  ellipse E104 centre (-8.625134, -25.663019) end of major axis (-9.3938, -25.441316) minor radius 0.14613 (-8.183521, -25.661407) -> (-8.415434, -25.57519) ccw
  ellipse E105 centre (-8.8976, -26.607686) end of major axis (-8.417184, -26.746251) minor radius 0.091331 (-8.738454, -26.741512) -> (-8.874319, -26.519348) ccw
  ellipse E106 centre (-8.8976, -26.607686) end of major axis (-8.128934, -26.829389) minor radius 0.14613 (-8.629467, -26.824599) -> (-8.5704, -26.561187) ccw
  line L142 (-8.128934, -26.829389) -> (-8.01781, -26.444112)
  ellipse E107 centre (-5.931589, -24.77436) end of major axis (-6.677372, -24.484865) minor radius 0.002457 (-6.623256, -24.504889) -> (-6.677372, -24.484865) ccw
  ellipse E108 centre (-5.931589, -24.77436) end of major axis (-5.185805, -25.063856) minor radius 0.002457 (-6.607137, -24.511015) -> (-6.609387, -24.510158) ccw
  line L143 (-4.546316, -25.309002) -> (-4.535532, -25.313185)
  line L144 (-4.535532, -25.313185) -> (-4.897399, -26.245409)
  ellipse E109 centre (-6.655324, -26.638809) end of major axis (-5.90954, -26.928305) minor radius 0.002457 (-6.364831, -26.753998) -> (-6.354481, -26.753176) ccw
  line L145 (-6.681027, -24.494282) -> (-6.677372, -24.484865)
  line L146 (-5.90954, -26.928305) -> (-5.550733, -26.003962)
  line L147 (-4.535532, -25.313185) -> (-4.519781, -25.272607)
  line L148 (-4.447272, -25.085815) -> (-2.532952, -20.154243)
  ellipse E110 centre (-4.747613, -25.984249) end of major axis (-3.855258, -25.591543) minor radius 0.168714 (-4.525819, -26.068175) -> (-3.856723, -25.623585) ccw
  line L149 (-3.856723, -25.623585) -> (-2.202821, -21.362887)
  line L150 (-4.525819, -26.068175) -> (-4.897399, -26.245409)
  line L151 (-4.897399, -26.245409) -> (-5.512305, -26.012732)
  line L152 (-5.475851, -26.021053) -> (-4.897399, -26.245409)
  ellipse E111 centre (-6.655324, -26.638809) end of major axis (-6.189209, -26.819744) minor radius 0.001536 (-6.362342, -26.753818) -> (-6.356896, -26.753385) ccw
  line L153 (5.3916, -24.802608) -> (6.669795, -24.558386)
  ellipse E112 centre (6.72089, -24.550899) end of major axis (7.506702, -24.400902) minor radius 0.002231 (6.869577, -24.520287) -> (6.669795, -24.558386) ccw
  ellipse E113 centre (6.72089, -24.550899) end of major axis (7.506702, -24.400902) minor radius 0.002231 (7.506702, -24.400902) -> (7.02461, -24.49083) ccw
  line L154 (7.507944, -24.407405) -> (7.506702, -24.400902)
  line L155 (8.131393, -24.534748) -> (9.071443, -24.429855)
  ellipse E114 centre (7.901177, -11.781775) end of major axis (9.394045, -11.63568) minor radius 0.24157 (9.328607, -11.57458) -> (9.230518, -11.544596) ccw
  ellipse E115 centre (7.901177, -11.781775) end of major axis (9.98124, -11.578215) minor radius 0.336587 (9.90778, -11.501324) -> (9.901805, -11.498416) ccw
  ellipse E116 centre (9.343058, -26.515593) end of major axis (8.845435, -26.564291) minor radius 0.080523 (8.909645, -26.517133) -> (8.859331, -26.542668) ccw
  ellipse E117 centre (9.343058, -26.515593) end of major axis (9.840681, -26.466894) minor radius 0.080523 (9.830382, -26.452729) -> (9.716254, -26.426506) ccw
  ellipse E118 centre (-6.707451, -24.57805) end of major axis (-5.922047, -24.730171) minor radius 0.086818 (-6.76123, -24.479557) -> (-7.355059, -24.404106) ccw
  line L156 (-6.76123, -24.479557) -> (-6.583025, -24.512275)
  line L157 (5.998893, -24.739555) -> (6.240444, -24.667892)
  ellipse E119 centre (6.28647, -24.656485) end of major axis (7.053465, -24.429067) minor radius 0.002152 (6.433133, -24.610796) -> (6.240444, -24.667892) ccw
  ellipse E120 centre (6.28647, -24.656485) end of major axis (7.053465, -24.429067) minor radius 0.002152 (6.504379, -24.589723) -> (6.50181, -24.590482) ccw
  ellipse E121 centre (6.28647, -24.656485) end of major axis (7.053465, -24.429067) minor radius 0.002152 (7.052921, -24.429145) -> (6.799543, -24.502689) ccw
  line L158 (5.017545, -26.073779) -> (4.918804, -25.740764)
  line L159 (2.991448, -18.539943) -> (2.981355, -18.542881)
  line L160 (3.734576, -21.74682) -> (2.886978, -18.888199)
  line L161 (5.028806, -26.070501) -> (5.017545, -26.073779)
  line L162 (5.017545, -26.073779) -> (4.953866, -26.03383)
  line L163 (5.017545, -26.073779) -> (5.248549, -26.005245)
  line L164 (8.589869, -24.510461) -> (8.607431, -24.506634)
  ellipse E122 centre (8.68203, -24.622177) end of major axis (9.46534, -24.45962) minor radius 0.128538 (8.84317, -24.461235) -> (8.607431, -24.506634) ccw
  line L165 (8.18773, -25.608236) -> (8.250937, -25.59446)
  ellipse E123 centre (9.083141, -26.555011) end of major axis (8.593572, -26.656609) minor radius 0.080336 (8.883698, -26.52039) -> (8.728163, -26.683203) ccw
  ellipse E124 centre (-9.604615, -24.525909) end of major axis (-10.404598, -24.53112) minor radius 0.125799 (-9.584414, -24.40002) -> (-10.404598, -24.53112) ccw
  line L166 (-9.584414, -24.40002) -> (-8.869777, -24.398319)
  line L167 (-8.031719, -24.396324) -> (-8.010084, -24.396273)
  line L168 (-8.010084, -24.396273) -> (-8.009893, -24.425527)
  ellipse E125 centre (-9.59175, -26.500985) end of major axis (-10.391733, -26.506196) minor radius 0.125799 (-9.306836, -26.381623) -> (-9.57155, -26.375096) ccw
  line L169 (-8.010084, -24.396273) -> (-8.013586, -23.858564)
  line L170 (-8.020128, -22.854147) -> (-8.023485, -22.338696)
  ellipse E126 centre (-9.694022, -10.799129) end of major axis (-11.783978, -10.812741) minor radius 0.328649 (-9.856288, -10.472496) -> (-10.885047, -10.536629) ccw
  ellipse E127 centre (-9.688233, -11.687913) end of major axis (-11.778189, -11.701526) minor radius 0.328649 (-9.932829, -11.36307) -> (-10.871432, -11.424514) ccw
  ellipse E128 centre (-9.688233, -11.687913) end of major axis (-11.188202, -11.697683) minor radius 0.235872 (-9.211723, -11.461228) -> (-11.185862, -11.710597) ccw
  ellipse E129 centre (-9.59175, -26.500985) end of major axis (-10.09174, -26.504242) minor radius 0.078624 (-9.707345, -26.425224) -> (-9.88676, -26.56634) ccw
  ellipse E130 centre (-7.178338, -24.486053) end of major axis (-7.975502, -24.418751) minor radius 0.002201 (-7.2621, -24.476785) -> (-7.975502, -24.418751) ccw
  line L171 (-7.976252, -24.427629) -> (-7.975502, -24.418751)
  line L172 (5.392589, -24.802419) -> (4.843658, -21.843171)
  line L173 (5.171436, -24.930004) -> (5.39714, -24.844259)
  line L174 (5.171436, -24.930004) -> (6.719114, -24.651335)
  ellipse E131 centre (6.74768, -24.567326) end of major axis (7.534262, -24.421417) minor radius 0.077504 (6.719114, -24.651335) -> (7.374646, -24.404547) ccw
  ellipse E132 centre (6.74768, -24.567326) end of major axis (5.961098, -24.713234) minor radius 0.077504 (7.372982, -24.404634) -> (7.367754, -24.404916) ccw
  line L175 (7.367754, -24.404916) -> (7.323464, -24.407369)
  line L176 (5.177718, -24.963873) -> (5.171436, -24.930004)
  line L177 (7.540538, -24.455255) -> (7.534262, -24.421417)
  line L178 (5.171436, -24.930004) -> (4.911774, -23.530187)
  line L179 (7.754227, -24.437676) -> (7.699555, -23.877595)
  line L180 (8.132564, -24.557058) -> (9.083915, -24.460121)
  ellipse E133 centre (9.14692, -24.500047) end of major axis (9.943136, -24.422325) minor radius 0.045982 (9.885218, -24.410919) -> (9.083915, -24.460121) ccw
  line L181 (7.500161, -24.401859) -> (7.45029, -23.890954)
  ellipse E134 centre (7.798741, -10.688671) end of major axis (9.878854, -10.485623) minor radius 0.120129 (9.865663, -10.473996) -> (9.104777, -10.467666) ccw
  ellipse E135 centre (7.886033, -11.582932) end of major axis (9.966146, -11.379885) minor radius 0.120129 (9.942069, -11.364581) -> (9.697526, -11.347367) ccw
  ellipse E136 centre (7.886033, -11.582932) end of major axis (9.378937, -11.437204) minor radius 0.086217 (9.224276, -11.491135) -> (9.215291, -11.414176) ccw
  ellipse E137 centre (9.340903, -26.487295) end of major axis (9.838538, -26.438719) minor radius 0.028739 (9.797345, -26.431384) -> (9.780884, -26.430998) ccw
  line L182 (-7.708273, -23.875552) -> (-7.762988, -24.435192)
  ellipse E138 centre (-9.139679, -24.498656) end of major axis (-9.935882, -24.420813) minor radius 0.045982 (-9.123008, -24.45409) -> (-9.877962, -24.409416) ccw
  line L183 (-9.123008, -24.45409) -> (-8.125158, -24.552534)
  ellipse E139 centre (-7.789398, -10.687485) end of major axis (-9.869481, -10.484121) minor radius 0.120129 (-9.0954, -10.466282) -> (-9.856288, -10.472496) ccw
  ellipse E140 centre (-7.876826, -11.581734) end of major axis (-9.956909, -11.37837) minor radius 0.120129 (-9.688283, -11.345892) -> (-9.932829, -11.36307) ccw
  ellipse E141 centre (-7.876826, -11.581734) end of major axis (-9.369709, -11.435779) minor radius 0.086217 (-9.206058, -11.412775) -> (-9.215056, -11.489733) ccw
  ellipse E142 centre (-9.333963, -26.485875) end of major axis (-8.836336, -26.534526) minor radius 0.028739 (-8.855298, -26.540413) -> (-8.876615, -26.519058) ccw
  ellipse E143 centre (-9.333963, -26.485875) end of major axis (-9.831591, -26.437223) minor radius 0.028739 (-9.613906, -26.434724) -> (-9.808187, -26.448418) ccw
  line L184 (-4.882738, -21.836972) -> (-5.427175, -24.769505)
  ellipse E144 centre (-6.740448, -24.5663) end of major axis (-7.527008, -24.420272) minor radius 0.077504 (-7.355059, -24.404106) -> (-6.816455, -24.630773) ccw
  line L185 (-6.816455, -24.630773) -> (-5.338013, -24.916966)
  line L186 (-7.53329, -24.454108) -> (-7.527008, -24.420272)
  line L187 (5.578671, -24.620574) -> (7.146042, -24.488271)
  ellipse E145 centre (7.185582, -24.487145) end of major axis (7.982757, -24.419965) minor radius 0.002201 (7.26771, -24.478027) -> (7.146042, -24.488271) ccw
  ellipse E146 centre (7.185582, -24.487145) end of major axis (7.982757, -24.419965) minor radius 0.002201 (7.982757, -24.419965) -> (7.267907, -24.478011) ccw
  line L188 (5.590804, -24.764547) -> (5.578671, -24.620574)
  line L189 (7.983505, -24.428843) -> (7.982757, -24.419965)
  line L190 (5.578671, -24.620574) -> (5.434593, -22.910918)
  line L191 (5.342219, -21.814792) -> (5.339729, -21.78525)
  line L192 (9.104977, -24.215504) -> (9.103856, -24.383719)
  line L193 (7.975779, -24.41203) -> (9.545121, -24.401574)
  ellipse E147 centre (9.611853, -24.52737) end of major axis (10.411835, -24.532703) minor radius 0.125799 (10.045396, -24.424463) -> (9.545121, -24.401574) ccw
  line L194 (7.975724, -24.420265) -> (7.975779, -24.41203)
  line L195 (7.975779, -24.41203) -> (7.979444, -23.862149)
  line L196 (7.986142, -22.857291) -> (7.991401, -22.068312)
  ellipse E148 centre (9.703348, -10.800604) end of major axis (7.613394, -10.786673) minor radius 0.328649 (10.894413, -10.538285) -> (9.865663, -10.473996) ccw
  ellipse E149 centre (9.697424, -11.689387) end of major axis (7.60747, -11.675457) minor radius 0.328649 (10.880662, -11.426168) -> (9.942069, -11.364581) ccw
  ellipse E150 centre (9.697424, -11.689387) end of major axis (11.19739, -11.699385) minor radius 0.235872 (11.179465, -11.73538) -> (9.220948, -11.46263) ccw
  ellipse E151 centre (9.60527, -25.514908) end of major axis (8.805288, -25.509575) minor radius 0.125799 (9.538539, -25.389111) -> (9.217186, -25.402378) ccw
  ellipse E152 centre (9.598688, -26.502445) end of major axis (10.098677, -26.505777) minor radius 0.078624 (9.951263, -26.448988) -> (9.714293, -26.426701) ccw
  line L197 (-8.191956, -25.598334) -> (-8.180328, -25.600757)
  ellipse E153 centre (-9.076212, -26.55363) end of major axis (-8.586658, -26.655302) minor radius 0.080336 (-8.721253, -26.681876) -> (-8.876764, -26.519039) ccw
  ellipse E154 centre (-6.279252, -24.65553) end of major axis (-7.046212, -24.427994) minor radius 0.002152 (-6.793616, -24.501269) -> (-7.045669, -24.428073) ccw
  line L198 (-3.482141, -20.54185) -> (-2.932828, -18.690261)
  line L199 (-2.973493, -18.54138) -> (-2.98297, -18.538642)
  ellipse E155 centre (7.900186, -22.030475) end of major axis (8.740777, -21.826434) minor radius 0.148059 (7.779215, -21.908284) -> (7.709154, -21.927158) ccw
  ellipse E156 centre (7.900186, -22.030475) end of major axis (8.740777, -21.826434) minor radius 0.148059 (7.969852, -21.862384) -> (7.922831, -21.872977) ccw
  ellipse E157 centre (-9.770217, -21.21726) end of major axis (-9.313361, -21.205783) minor radius 0.076505 (-9.390136, -21.165517) -> (-9.943174, -21.15065) ccw
  ellipse E158 centre (-9.770217, -21.21726) end of major axis (-10.634944, -21.238982) minor radius 0.144806 (-9.26864, -21.087019) -> (-10.477115, -21.317948) ccw
  ellipse E159 centre (-9.794975, -20.231682) end of major axis (-10.659703, -20.253405) minor radius 0.144806 (-9.577407, -20.086179) -> (-10.659703, -20.253405) ccw
  line L200 (-10.659703, -20.253405) -> (-10.634944, -21.238982)
  ellipse E160 centre (-7.054088, -21.957117) end of major axis (-7.916875, -21.895274) minor radius 0.002538 (-6.95652, -21.961583) -> (-7.700808, -21.912446) ccw
  line L201 (-7.887515, -21.485673) -> (-7.916875, -21.895274)